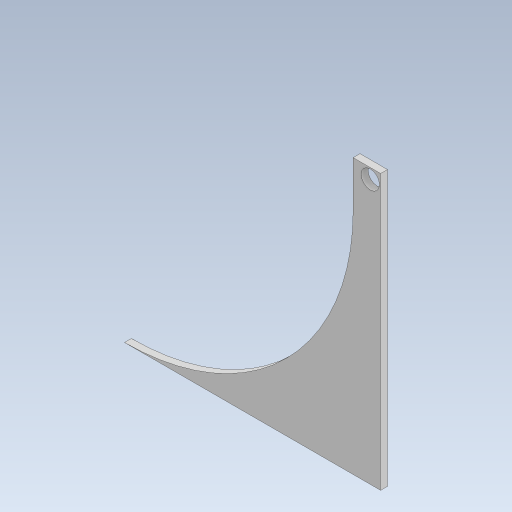
# Autodesk Inventor part: 零件10
Saved by Autodesk Inventor 2023 (Build 270158000, 158)
## iProperties
Created: 2023-05-16
Part Number: 零件10
Material: 一般
Document SubType Name: Modeling
Designer: Johnny Jou
Density: 1 g/cm^3
Appearance: 預設
Author: Johnny Jou
Autodesk Inventor part; units mm, degrees
ref_plane "YZ Plane" through (0, 0, 0) normal (1, 0, 0) x (0, 1, 0)
ref_plane "XZ Plane" through (0, 0, 0) normal (0, 1, 0) x (-1, 0, 0)
ref_plane "XY Plane" through (0, 0, 0) normal (0, 0, 1) x (1, 0, 0)
sketch "草圖1" plane through (0, 0, 0) normal (0, 0, 1) x (1, 0, 0)
  line L0 (0, -80) -> (100, -80)
  arc A0 (100, -80) -> (200, 20) centre (100, 20) ccw
  line L1 (200, 20) -> (200, 40)
  line L2 (200, 40) -> (100, 40)
  line L3 (100, 40) -> (100, -80)
  line L4 (100, -80) -> (200, -80)
  line L5 (200, -80) -> (200, 40)
  line L6 (200, 40) -> (212, 40)
  line L7 (212, 40) -> (212, -80)
  line L8 (212, -80) -> (200, -80)
  line L9 (200, -80) -> (200, 40)
  circle A1 centre (207.5, 35.5) radius 4
  point P0 (200, 20)
  point P1 (200, 20)
  dimension "d0" = 8
  dimension "d4" = 4.5
  dimension "d5" = 4.5
  constraints: 20 end point, 4 parallel, 3 horizontal, 2 centre point, 2 perpendicular, 2 point on circle, 1 collinear, 1 vertical, 5 other
  measures "d0" diameter of A1
  measures "d4" distance from line of L6 A1.centre
  measures "d5" distance from line of L7 A1.centre
extrude "擠出1" add sketch "草圖1" along normal blind 3 contours A0 L5 L4 | L1 L6 L7 L8 L5
